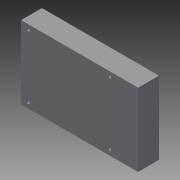
# Autodesk Inventor part: orangepi
Saved by Autodesk Inventor 2013 (Build 170138000, 138)
## iProperties
Created: 2015-06-07
Part Number: orangepi
Material: Generic
Document SubType Name: Modeling
Designer: Jufo
Density: 1 g/cm^3
Author: Jufo
Autodesk Inventor part; units mm, degrees
ref_plane "YZ Plane" through (0, 0, 0) normal (1, 0, 0) x (0, 1, 0)
ref_plane "XZ Plane" through (0, 0, 0) normal (0, 1, 0) x (-1, 0, 0)
ref_plane "XY Plane" through (0, 0, 0) normal (0, 0, 1) x (1, 0, 0)
sketch "Sketch1" plane through (0, 0, 0) normal (0, 1, 0) x (-1, 0, 0)
  line L0 (-27.4703, 30.0521) -> (73.5297, 30.0521)
  line L1 (73.5297, 30.0521) -> (73.5297, -32.9479)
  line L2 (73.5297, -32.9479) -> (-27.4703, -32.9479)
  line L3 (-27.4703, -32.9479) -> (-27.4703, 30.0521)
  circle A0 centre (67.4297, 26.1521) radius 1.5
  circle A1 centre (67.4297, -28.0479) radius 1.5
  circle A2 centre (-2.7703, 26.1521) radius 1.5
  circle A3 centre (-2.7703, -28.0479) radius 1.5
  point P0 (0, 0)
  dimension "d0" = 101
  dimension "d2" = 63
  dimension "d3" = 3
  dimension "d4" = 3
  dimension "d5" = 3
  dimension "d6" = 3
  dimension "d9" = 3.9
  dimension "d10" = 3.9
  dimension "d11" = 6.1
  dimension "d12" = 70.2
  dimension "d14" = 6.1
  dimension "d15" = 70.2
  dimension "d18" = 54.2
  dimension "d19" = 54.2
  constraints: 8 end point, 4 centre point, 2 parallel, 1 horizontal, 1 perpendicular
  measures "d0" distance of L0.start L0.end
  measures "d2" distance of L0.end L1.end
  measures "d3" diameter of A0
  measures "d4" diameter of A2
  measures "d5" diameter of A3
  measures "d6" diameter of A1
  measures "d9" distance from line of L0 A2.centre
  measures "d10" distance from line of L0 A0.centre
  measures "d11" distance from line of L1 A0.centre
  measures "d12" distance of A2.centre A0.centre
  measures "d14" distance from line of L1 A1.centre
  measures "d15" distance of A1.centre A3.centre
  measures "d18" distance of A1.centre A0.centre
  measures "d19" distance of A3.centre A2.centre
extrude "Extrusion1" add sketch "Sketch1" along normal blind 18
body "Solid1"
